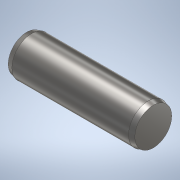
# Autodesk Inventor part: φ4ピン　L20
Saved by Autodesk Inventor 2020 (Build 240168000, 168)
## iProperties
Part Number: φ4ピン　L20
Material: ステンレス鋼
Document SubType Name: Modeling
Designer: 原知也
Density: 8 g/cm^3
Appearance: 半つや出し
Mass: 2.00023 g
Surface Area: 2.72263 cm^2
Volume: 0.250029 cm^3
Author: 原知也
Autodesk Inventor part; units mm, degrees
ref_plane "YZ Plane" through (0, 0, 0) normal (1, 0, 0) x (0, 1, 0)
ref_plane "XZ Plane" through (0, 0, 0) normal (0, 1, 0) x (-1, 0, 0)
ref_plane "XY Plane" through (0, 0, 0) normal (0, 0, 1) x (1, 0, 0)
sketch "スケッチ1" plane through (0, 0, 0) normal (0, 0, 1) x (1, 0, 0)
  line L0 (-18.9602, 2.8145) -> (-4.2202, 2.8145)
  line L1 (-3.5902, 2.6457) -> (-3.5902, 0.3145)
  line L2 (-19.5902, 0.3145) -> (-19.5902, 2.6457)
  line L3 (-18.9602, 2.8145) -> (-18.9602, -1.1855) construction
  line L4 (-4.2202, 2.8145) -> (-4.2202, -1.1855) construction
  line L5 (-18.9602, 2.8145) -> (-19.5902, 2.6457)
  line L6 (-4.2202, 2.8145) -> (-3.5902, 2.6457)
  line L7 (-35.0163, 0.3145) -> (16.7265, 0.3145) construction
  line L8 (-19.5902, 0.3145) -> (-3.5902, 0.3145)
  dimension "d2" = 0.63
  dimension "d3" = 0.63
  dimension "d4" = 15
  dimension "d6" = 15
  dimension "d9" = 16
  dimension "d12" = 2.5
  constraints: 18 end point, 3 horizontal, 2 point on line, 1 parallel, 1 perpendicular
  measures "d2" distance between parallel lines of L3 L2
  measures "d3" distance between parallel lines of L1 L4
  measures "d4" angle of L5 L0
  measures "d6" angle of L0 L6
  measures "d9" distance between parallel lines of L2 L1
  measures "d12" distance between parallel lines of L7 L0
revolve "回転1" add sketch "スケッチ1" angle 360 about axis through (-35.0163, 0.3145, 0) along (1, 0, 0)
